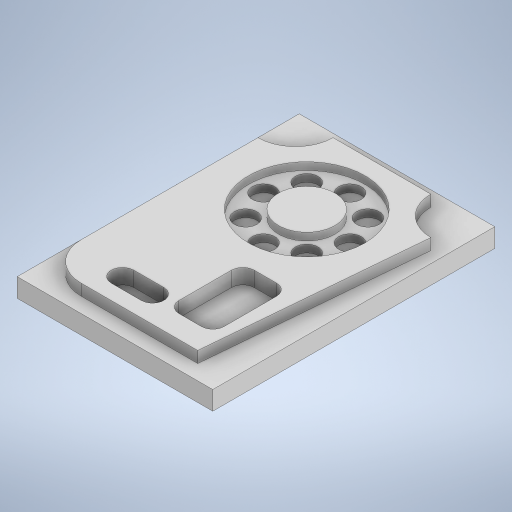
# Autodesk Inventor part: A2P2
Saved by Autodesk Inventor 2023.2 (Build 272271000, 271)
## iProperties
Created: 2023-01-23
Part Number: A2P2
Material: Generic
Document SubType Name: Modeling
Designer: manas
Density: 1 g/cm^3
Appearance: Default
Author: manas
Autodesk Inventor part; units mm, degrees
ref_plane "YZ Plane" through (0, 0, 0) normal (1, 0, 0) x (0, 1, 0)
ref_plane "XZ Plane" through (0, 0, 0) normal (0, 1, 0) x (-1, 0, 0)
ref_plane "XY Plane" through (0, 0, 0) normal (0, 0, 1) x (1, 0, 0)
sketch "Sketch1" plane through (0, 0, 0) normal (0, 1, 0) x (-1, 0, 0)
  line L0 (26, 37.5) -> (-26, 37.5)
  line L1 (-26, 37.5) -> (-26, -37.5)
  line L2 (-26, -37.5) -> (26, -37.5)
  line L3 (26, -37.5) -> (26, 37.5)
  line L4 (26, 37.5) -> (-26, -37.5) construction
  line L5 (-26, 37.5) -> (26, -37.5) construction
  point P0 (0, 0)
  dimension "d0" = 52
  dimension "d1" = 75
  constraints: 12 end point, 2 midpoint, 2 parallel, 1 horizontal, 1 perpendicular
  measures "d0" distance of L2.end L1.end
  measures "d1" distance of L1.end L0.end
extrude "Extrusion1" add sketch "Sketch1" along normal blind 5
sketch "Sketch2" plane through (0, 5, 0) normal (0, 1, 0) x (1, 0, 0)
  line L0 (-13, -33.5) -> (35.879, -33.5)
  line L1 (-26, -37.5) -> (26, -37.5) projected
  line L2 (-23, -23.5) -> (-23, 74.0013)
  line L3 (-26, 37.5) -> (-26, -37.5) projected
  arc A0 (-23, 23.5) -> (-13, 33.5) centre (-23, 33.5) ccw
  line L4 (26, 37.5) -> (-26, 37.5) projected
  arc A1 (13, 33.5) -> (23, 23.5) centre (23, 33.5) ccw
  line L5 (26, -37.5) -> (26, 37.5) projected
  line L6 (-13, 33.5) -> (13, 33.5)
  line L7 (18, -33.5) -> (23, 23.5)
  arc A2 (-23, -23.5) -> (-13, -33.5) centre (-13, -23.5) ccw
  point P0 (0, 0)
  dimension "d4" = 4
  dimension "d5" = 3
  dimension "d6" = 20
  dimension "d7" = 4
  dimension "d8" = 20
  dimension "d9" = 4
  dimension "d10" = 3
  dimension "d11" = 8
  dimension "d12" = 3
  dimension "d13" = 10
  constraints: 8 end point, 6 point on circle, 3 centre point, 3 point on line, 2 horizontal, 2 tangent, 1 vertical
  measures "d4" distance between parallel lines of L1 L0
  measures "d5" distance between parallel lines of L3 L2
  measures "d6" diameter of A0
  measures "d7" distance from line of L4 A0.centre
  measures "d8" diameter of A1
  measures "d9" distance from line of L4 A1.centre
  measures "d10" distance from line of L5 A1.centre
  measures "d11" distance from line of L5 L7.start
  measures "d12" distance from line of L7.end L5
  measures "d13" radius of A2
extrude "Extrusion2" add sketch "Sketch2" along normal blind 3 contours A2 L2 A0 L6 A1 L7 L0
sketch "Sketch3" plane through (0, 8, 0) normal (0, 1, 0) x (1, 0, 0)
  line L0 (4, -10.5) -> (4, -24.5)
  line L1 (7, -27.5) -> (13, -27.5)
  line L2 (16, -24.5) -> (16, -10.5)
  line L3 (13, -7.5) -> (7, -7.5)
  line L4 (26, -37.5) -> (26, 37.5) projected
  line L5 (-26, -37.5) -> (26, -37.5) projected
  arc A0 (4, -24.5) -> (7, -27.5) centre (7, -24.5) ccw
  arc A1 (7, -7.5) -> (4, -10.5) centre (7, -10.5) ccw
  arc A2 (16, -10.5) -> (13, -7.5) centre (13, -10.5) ccw
  arc A3 (13, -27.5) -> (16, -24.5) centre (13, -24.5) ccw
  arc A4 (-9, -23.5) -> (-9, -29.5) centre (-9, -26.5) ccw
  arc A5 (-1, -29.5) -> (-1, -23.5) centre (-1, -26.5) ccw
  line L6 (-9, -23.5) -> (-1, -23.5)
  line L7 (-9, -29.5) -> (-1, -29.5)
  circle A6 centre (0, 13.5) radius 7.5
  circle A7 centre (0, 2) radius 3
  circle A8 centre (-8.1317, 5.3683) radius 3
  circle A9 centre (-11.5, 13.5) radius 3
  circle A10 centre (-8.1317, 21.6317) radius 3
  circle A11 centre (0, 25) radius 3
  circle A12 centre (8.1317, 21.6317) radius 3
  circle A13 centre (11.5, 13.5) radius 3
  circle A14 centre (8.1317, 5.3683) radius 3
  point P0 (0, 0)
  point P1 (4, -7.5)
  point P2 (4, -27.5)
  point P3 (16, -27.5)
  dimension "d16" = 22
  dimension "d17" = 30
  dimension "d18" = 20
  dimension "d19" = 12
  dimension "d20" = 3
  dimension "d21" = 6
  dimension "d22" = 6
  dimension "d23" = 27
  dimension "d24" = 11
  dimension "d25" = 11
  dimension "d26" = 35
  dimension "d27" = 15
  dimension "d28" = 51
  dimension "d29" = 26
  dimension "d30" = 6
  dimension "d31" = 11.5
  dimension "d34" = 360
  constraints: 15 centre point, 12 end point, 12 point on circle, 10 tangent, 6 point on line, 3 equal radius, 2 coincident, 2 horizontal, 2 parallel, 1 perpendicular, 1 vertical, 23 other
  measures "d16" distance between parallel lines of L4 L0
  measures "d17" distance between parallel lines of L5 L3
  measures "d18" distance of point (4, -7.5) point (4, -27.5)
  measures "d19" distance of point (4, -27.5) point (16, -27.5)
  measures "d20" radius of A0
  measures "d21" diameter of A4
  measures "d22" diameter of A5
  measures "d23" distance from line of L4 A5.centre
  measures "d24" distance from line of L5 A5.centre
  measures "d25" distance from line of L5 A4.centre
  measures "d26" distance from line of L4 A4.centre
  measures "d27" diameter of A6
  measures "d28" distance from line of L5 A6.centre
  measures "d29" distance from line of L4 A6.centre
  measures "d30" diameter of A7
  measures "d31" distance of A7.centre A6.centre
extrude "Extrusion3" cut sketch "Sketch3" against normal blind 4 contours A1 L3 A2 L2 A3 L1 A0 L0 | L6 A5 L7 A4 | A7 | A8 | A9 | A10 | A11 | A12 | A13 | A14
sketch "Sketch4" plane through (0, 8, 0) normal (0, 1, 0) x (1, 0, 0)
  circle A0 centre (0, 13.5) radius 7.5
  line L0 (26, -37.5) -> (26, 37.5) projected
  line L1 (-26, -37.5) -> (26, -37.5) projected
  circle A1 centre (0, 13.5) radius 15.5
  point P0 (0, 0)
  dimension "d38" = 15
  dimension "d39" = 26
  dimension "d40" = 51
  dimension "d41" = 31
  constraints: 2 centre point, 1 coincident
  measures "d38" diameter of A0
  measures "d39" distance from line of L0 A0.centre
  measures "d40" distance from line of L1 A0.centre
  measures "d41" diameter of A1
extrude "Extrusion4" cut sketch "Sketch4" against normal blind 2
body "Solid1"
